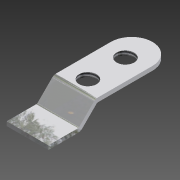
# Autodesk Inventor part: Blaszka_do_ciągu
Saved by Autodesk Inventor 2015 (Build 190159000, 159)
## iProperties
Created: 2016-01-12
Part Number: Blaszka_do_ciągu
Material: Aluminium 6061-AHC
Document SubType Name: Modelowanie
Designer: graaapsik
Density: 2.71 g/cm^3
Appearance: Aluminium - ciemne
Sheet Metal Rule: Default
Mass: 6.01462 g
Surface Area: 26.4007 cm^2
Volume: 2.21942 cm^3
Author: graaapsik
Autodesk Inventor part; units mm, degrees
ref_plane "YZ Plane" through (0, 0, 0) normal (1, 0, 0) x (0, 1, 0)
ref_plane "XZ Plane" through (0, 0, 0) normal (0, 1, 0) x (-1, 0, 0)
ref_plane "XY Plane" through (0, 0, 0) normal (0, 0, 1) x (1, 0, 0)
sketch "Szkic1" plane through (0, 0, 0) normal (0, 1, 0) x (-1, 0, 0)
  line L0 (0, 0) -> (20, 0)
  line L1 (20, 0) -> (20, 2)
  line L2 (20, 2) -> (0, 2)
  line L3 (0, 2) -> (0, 0)
  dimension "d20" = 20
  dimension "d21" = 2
  constraints: 8 end point, 2 parallel, 1 horizontal, 1 perpendicular
  measures "d20" distance of L0.start L0.end
  measures "d21" distance of L0.end L1.end
sketch "Szkic5" plane through (0, 0, 0) normal (1, 0, 0) x (0, 1, 0)
  line L0 (0, 2) -> (0, 0) construction
  line L1 (0, 1) -> (14.1716, 1)
  line L2 (15.5858, 1.5858) -> (22.4142, 8.4142)
  line L3 (23.8284, 9) -> (60, 9)
  arc A0 (14.1716, 1) -> (15.5858, 1.5858) centre (14.1716, 3) ccw
  arc A1 (23.8284, 9) -> (22.4142, 8.4142) centre (23.8284, 7) ccw
  point P0 (15, 1)
  point P1 (23, 9)
  dimension "d22" = 15
  dimension "d23" = 8
  dimension "d24" = 60
  dimension "d25" = 45
  dimension "d27" = 2
  constraints: 6 end point, 4 point on circle, 4 point on line, 4 tangent, 2 centre point, 1 equal radius, 1 midpoint, 1 parallel, 1 perpendicular
  measures "d22" distance of L1.start point (15, 1)
  measures "d23" distance between parallel lines of L1 L3
  measures "d24" horizontal distance of L1.start L3.end
  measures "d25" angle of L3 L2
  measures "d27" radius of A0
sweep "Przeciągnięcie1" add profiles "Szkic1" path "Szkic5" path curves L1 A0 L2 A1 L3
fillet "Zaokrąglenie1" radius 10 2 edges at (-20, 60, 9) (0, 60, 9)
sketch "Szkic2" plane through (-20, 23.8284, 10) normal (0, 0, 1) x (1, 0, 0)
  arc A0 (20, 26.1716) -> (0, 26.1716) centre (10, 26.1716) ccw projected
  point P0 (10, 23.1716)
  dimension "d29" = 3
  constraints: 1 vertical alignment
  measures "d29" distance of A0.centre point (10, 23.172)
hole "Otwór1" at (-10, 47, 10) direction (0, 0, -1) diameter 8.376 end through all
pattern_linear "Szyk prostokątny2" count 2 spacing 18 along (0, -1, 0) of "Otwór1"
equation "\"d12\" = Grubość"
equation "\"PromieńGięcia\" = Grubość"
equation "\"SzerokośćGięciaPodcięcia\" = Grubość"
equation "\"GłębokośćGięciaPodcięcia\" = 0.5 * Grubość"
equation "\"RozmiarPodcięciaNarożnika\" = 4 * Grubość"
equation "\"MinimalnaPozostałość\" = 2 * Grubość"
equation "\"PromieńPrzejścia\" = PromieńGięcia"
equation "\"Rozmiar_promienia_Jacobiego\" = Grubość"
equation "\"Wielk_odstępu\" = Grubość"
equation "\"d5\" = PromieńGięcia"
equation "\"Grubość\" = 2"
